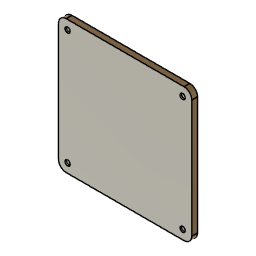
bottom_access_panel (Autodesk Fusion 360 design; units mm, degrees)
Autodesk Fusion 360 part; units mm, degrees
sketch "Bottom Access Panel" plane through (0, 0, 0) normal (0, 1, 0) x (1, 0, 0)
  line L0 (0, 0) -> (139, 0)
  line L1 (139, 0) -> (139, -139)
  line L2 (139, -139) -> (0, -139)
  line L3 (0, -139) -> (0, 0)
  dimension "d1" = 139
  dimension "d2" = 139
  constraint horizontal L0
  constraint vertical L1
  constraint horizontal L2
  constraint vertical L3
  constraint coincident L0.start L3.end
  measures "d1" distance of L0.start L0.end
  measures "d2" distance of L0.end L1.end
extrude "Extrude1" add sketch "Bottom Access Panel" along normal blind 6
fillet "Fillet1" radius 8 4 edges at (0, 3, 139) (139, 3, 139) (139, 3, 0) (0, 3, 0)
sketch "Magnet Holes" plane through (0, 0, 0) normal (0, 1, 0) x (1, 0, 0)
  arc A0 (8, 0) -> (0, -8) centre (8, -8) ccw
  line L0 (8, 0) -> (131, 0)
  arc A1 (139, -8) -> (131, 0) centre (131, -8) ccw
  line L1 (139, -8) -> (139, -131)
  arc A2 (131, -139) -> (139, -131) centre (131, -131) ccw
  line L2 (131, -139) -> (8, -139)
  arc A3 (0, -131) -> (8, -139) centre (8, -131) ccw
  line L3 (0, -131) -> (0, -8)
  circle A4 centre (9.5, -129.5) radius 2.75
  circle A5 centre (129.5, -129.5) radius 2.75
  circle A6 centre (9.5, -9.5) radius 2.75
  circle A7 centre (129.5, -9.5) radius 2.75
  dimension "d20" = 5.5
  dimension "d21" = 5.5
  dimension "d22" = 5.5
  dimension "d23" = 5.5
  dimension "d24" = 9.5
  dimension "d25" = 9.5
  dimension "d26" = 9.5
  dimension "d27" = 9.5
  dimension "d28" = 9.5
  dimension "d29" = 9.5
  dimension "d30" = 9.5
  dimension "d31" = 9.5
  measures "d20" diameter of A4
  measures "d21" diameter of A5
  measures "d22" diameter of A6
  measures "d23" diameter of A7
  measures "d24" distance of L1 A5.centre
  measures "d25" distance of L2 A5.centre
  measures "d26" distance of L3 A4.centre
  measures "d27" distance of L2 A4.centre
  measures "d28" distance of L0 A6.centre
  measures "d29" distance of L3 A6.centre
  measures "d30" distance of L1 A7.centre
  measures "d31" distance of L0 A7.centre
extrude "Extrude3" cut sketch "Magnet Holes" along normal blind 1.5 contours A4 | A5 | A6 | A7
equation "mdfThickness = 6 mm" comment "Thickness of the MDF fibre board"
equation "d4 = mdfThickness"
equation "filletRadius = 8 mm" comment "Radius to use for fillets"
equation "d15 = filletRadius"
named bodies: "Bottom Access Panel"
